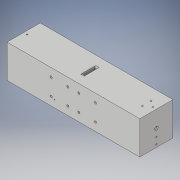
# Autodesk Inventor part: block
Saved by Autodesk Inventor 2017 (Build 210142000, 142)
## iProperties
Created: 2017-11-18
Part Number: block
Material: Generic
Document SubType Name: Modeling
Designer: Andy
Density: 1 g/cm^3
Appearance: Default
Author: Andy
Autodesk Inventor part; units mm, degrees
ref_plane "YZ Plane" through (0, 0, 0) normal (1, 0, 0) x (0, 1, 0)
ref_plane "XZ Plane" through (0, 0, 0) normal (0, 1, 0) x (-1, 0, 0)
ref_plane "XY Plane" through (0, 0, 0) normal (0, 0, 1) x (1, 0, 0)
sketch "Sketch1" plane through (0, 0, 0) normal (0, 0, 1) x (1, 0, 0)
  line L0 (-395.4763, 28.0534) -> (214.1237, 28.0534)
  line L1 (214.1237, 28.0534) -> (214.1237, -124.3466)
  line L2 (214.1237, -124.3466) -> (-395.4763, -124.3466)
  line L3 (-395.4763, -124.3466) -> (-395.4763, 28.0534)
  line L4 (100.4888, 124.4295) -> (100.4888, 286.3545)
  line L5 (100.4888, 286.3545) -> (135.4138, 286.3545)
  line L6 (137.9237, 286.3545) -> (137.9237, 124.4295)
  line L7 (137.9237, 124.4295) -> (100.4888, 124.4295)
  point P0 (0, 0)
  dimension "d0" = 609.6
  dimension "d1" = 152.4
  dimension "d7" = 161.925
  dimension "d8" = 34.925
  constraints: 16 end point, 3 perpendicular, 2 parallel, 2 vertical, 1 horizontal, 1 point on line
  measures "d0" distance between parallel lines of L1 L3
  measures "d1" distance between parallel lines of L2 L0
  measures "d7" distance of L4.start L4.end
  measures "d8" distance of L4.end L5.end
extrude "Extrusion1" add sketch "Sketch1" along normal blind 152.4
sketch "Sketch4" plane through (214.1237, -124.3466, 0) normal (1, 0, 0) x (0, 0, -1)
  circle A0 centre (-76.2, 76.2) radius 5.1594
  line L0 (-152.4, 0) -> (-152.4, 152.4) projected
  line L1 (0, 152.4) -> (-152.4, 152.4) projected
  point P0 (0, 124.3466)
  dimension "d1" = 152.4
  dimension "d9" = 10.3187
  constraints: 1 centre point
  measures "d9" diameter of A0
extrude "Extrusion2" cut sketch "Sketch4" against normal blind 609.6
sketch "Sketch5" plane through (-395.4763, 28.0534, 0) normal (0, 1, 0) x (1, 0, 0)
  line L0 (609.6, -152.4) -> (0, -152.4) projected
  line L1 (0, -152.4) -> (0, 0) projected
  line L2 (0, 0) -> (609.6, 0) projected
  line L3 (609.6, 0) -> (609.6, -152.4) projected
  line L4 (609.6, -152.4) -> (0, -152.4) projected
  line L5 (609.6, 0) -> (609.6, -152.4) projected
  line L6 (0, 0) -> (0, -152.4) projected
  line L7 (0, 0) -> (609.6, 0) projected
  line L8 (297.18, -104.775) -> (312.42, -104.775)
  line L9 (312.42, -104.775) -> (312.42, -47.625)
  line L10 (312.42, -47.625) -> (297.18, -47.625)
  line L11 (297.18, -47.625) -> (297.18, -104.775)
  line L12 (297.18, -104.775) -> (312.42, -47.625) construction
  line L13 (312.42, -104.775) -> (297.18, -47.625) construction
  point P0 (395.4763, 0)
  point P1 (297.0135, -78.1466)
  point P2 (312.2535, -78.0634)
  point P3 (312.2535, -74.3366)
  point P4 (304.8, -76.2)
  dimension "d1" = 152.4
  dimension "d48" = 15.24
  dimension "d49" = 57.15
  dimension "d50" = 47.625
  dimension "d51" = 47.625
  constraints: 12 end point, 2 midpoint, 2 parallel, 1 horizontal, 1 perpendicular
  measures "d48" distance of L10.end L9.end
  measures "d49" distance between parallel lines of L8 L10
  measures "d50" distance between parallel lines of L2 L10
  measures "d51" distance between parallel lines of L0 L8
extrude "Extrusion3" cut sketch "Sketch5" against normal blind 609.6 contours L11 L10 L9 L8
fillet "Fillet1" radius 6.35 4 edges at (-90.6763, 28.0534, 47.625) (-90.6763, 28.0534, 104.775) (-90.6763, -124.3466, 47.625) (-90.6763, -124.3466, 104.775)
chamfer "Chamfer1" distance 3.175 angle 45 1 edges at (214.1237, -48.1466, 81.3594) measured on face at (16.0037, -48.5618, 71.0574)
chamfer "Chamfer2" distance 3.175 angle 45 1 edges at (-395.4763, -48.1466, 81.3594) measured on face at (-296.4163, -48.5618, 71.0574)
sketch "Sketch6" plane through (-395.4763, 28.0534, 0) normal (0, 1, 0) x (1, 0, 0)
  line L0 (609.6, 0) -> (609.6, -152.4) projected
  line L1 (609.6, -152.4) -> (0, -152.4) projected
  line L2 (0, -152.4) -> (0, 0) projected
  line L3 (0, 0) -> (609.6, 0) projected
  line L4 (609.6, -84.5344) -> (609.6, -67.8656) projected
  line L5 (609.6, -76.2) -> (625.475, -76.2) construction
  circle A0 centre (593.725, -76.2) radius 3.175
  line L6 (0, 0) -> (0, -152.4) projected
  circle A1 centre (15.875, -76.2) radius 3.175
  line L7 (297.18, -41.275) -> (312.42, -41.275) projected
  line L8 (312.42, -111.125) -> (312.42, -41.275) projected
  line L9 (312.42, -111.125) -> (297.18, -111.125) projected
  line L10 (297.18, -41.275) -> (297.18, -111.125) projected
  point P0 (395.4763, 0)
  dimension "d1" = 152.4
  dimension "d30" = 6.35
  dimension "d34" = 6.35
  constraints: 2 centre point, 2 end point, 1 horizontal, 1 midpoint
  measures "d30" diameter of A0
  measures "d34" diameter of A1
extrude "Extrusion4" cut sketch "Sketch6" against normal blind 101.6 contours A0 | A1
sketch "Sketch7" plane through (-395.4763, 28.0534, 0) normal (0, 1, 0) x (1, 0, 0)
  circle A0 centre (593.725, -76.2) radius 3.175 construction
  circle A1 centre (15.875, -76.2) radius 3.175 projected
  line L0 (609.6, 0) -> (609.6, -152.4) construction
  line L1 (609.6, -152.4) -> (0, -152.4) projected
  line L2 (0, -152.4) -> (0, 0) projected
  line L3 (0, 0) -> (609.6, 0) projected
  line L4 (609.6, -152.4) -> (0, -152.4) projected
  line L5 (565.15, -152.4) -> (565.15, 0) construction
  line L6 (609.6, 0) -> (609.6, -152.4) construction
  line L7 (297.18, -41.275) -> (312.42, -41.275) projected
  line L8 (312.42, -111.125) -> (312.42, -41.275) projected
  line L9 (312.42, -111.125) -> (297.18, -111.125) projected
  line L10 (297.18, -41.275) -> (297.18, -111.125) projected
  line L11 (609.6, -76.2) -> (629.3437, -76.2) construction
  line L12 (629.3437, -56.1975) -> (609.6, -56.1975) construction
  line L13 (629.3437, -96.2025) -> (609.6, -96.2025) construction
  line L14 (609.6, -96.2025) -> (529.5756, -96.2025) construction
  line L15 (609.6, -56.1975) -> (531.5543, -56.1975) construction
  circle A2 centre (565.15, -96.2025) radius 3.175
  circle A3 centre (565.15, -56.1975) radius 3.175
  point P0 (395.4763, 0)
  dimension "d1" = 152.4
  dimension "d37" = 44.45
  dimension "d85" = 20.0025
  dimension "d86" = 40.005
  dimension "d87" = 6.35
  dimension "d88" = 6.35
  dimension "d89" = 44.45
  constraints: 12 end point, 6 point on line, 3 horizontal, 2 centre point, 1 midpoint, 1 vertical
  measures "d37" distance between parallel lines of L5 L0
  measures "d85" distance between parallel lines of L11 L12
  measures "d86" distance between parallel lines of L12 L13
  measures "d87" diameter of A2
  measures "d88" diameter of A3
  measures "d89" distance from line of A2.centre L0
extrude "Extrusion5" cut sketch "Sketch7" against normal blind 28.575 contours A2 | A3
sketch "Sketch9" plane through (-395.4763, -124.3466, 0) normal (0, -1, 0) x (1, 0, 0)
  line L0 (609.6, 152.4) -> (609.6, 0) projected
  line L1 (609.6, 0) -> (0, 0) projected
  line L2 (0, 0) -> (0, 152.4) projected
  line L3 (0, 152.4) -> (609.6, 152.4) projected
  line L4 (312.42, 41.275) -> (297.18, 41.275) projected
  line L5 (297.18, 111.125) -> (297.18, 41.275) projected
  line L6 (297.18, 111.125) -> (312.42, 111.125) projected
  line L7 (312.42, 41.275) -> (312.42, 111.125) projected
  line L8 (0, 76.2) -> (609.6, 76.2) construction
  circle A0 centre (218.44, 76.2) radius 19.685
  point P0 (395.4763, 0)
  dimension "d1" = 152.4
  dimension "d65" = 39.37
  dimension "d66" = 78.74
  dimension "d69" = 0
  constraints: 2 end point, 2 midpoint, 1 centre point
  measures "d65" diameter of A0
  measures "d66" distance from line of L5 A0.centre
  measures "d69" distance from line of L8 A0.centre
extrude "Extrusion8" cut sketch "Sketch9" against normal blind 63.5 contours A0
sketch "Sketch10" plane through (0, 0, 152.4) normal (0, 0, 1) x (1, 0, 0)
  line L0 (214.1237, 28.0534) -> (214.1237, -124.3466) projected
  line L1 (214.1237, -124.3466) -> (-395.4763, -124.3466) projected
  line L2 (-395.4763, -124.3466) -> (-395.4763, 28.0534) projected
  line L3 (-395.4763, 28.0534) -> (214.1237, 28.0534) projected
  line L4 (-157.3513, -124.3466) -> (-196.7213, -124.3466) projected
  line L5 (-157.3513, -60.8466) -> (-196.7213, -60.8466) projected
  line L6 (-157.3513, -124.3466) -> (-196.7213, -124.3466) projected
  line L7 (-157.3513, -92.075) -> (-196.7213, -92.075)
  line L8 (-177.0363, -92.075) -> (-177.0363, -60.8466)
  point P0 (0, 0)
  dimension "d1" = 152.4
  dimension "d72" = 31.2284
  constraints: 4 end point, 2 midpoint, 1 parallel
  measures "d72" distance between parallel lines of L5 L7
hole "Hole1" at (-177.0363, -92.075, 152.4) direction (0, 0, -1) diameter 3.9624 depth 13.6144 tip angle 118 thread size "10-32 UNF" class "2B" standard "ANSI Unified Screw Threads"
sketch "Sketch11" plane through (214.1237, -124.3466, 0) normal (1, 0, 0) x (0, 0, -1)
  circle A0 centre (-76.2, 12.7) radius 3.175 projected
  circle A1 centre (-76.2, 42.0133) radius 3.175 projected
  point P0 (0, 124.3466)
  dimension "d1" = 152.4
extrude "Extrusion9" cut sketch "Sketch11" against normal blind 28.575
thread "Thread7" size "1/4-20 UNC" class "2B" standard "ANSI Unified Screw Threads" full length
thread "Thread8" size "1/4-20 UNC" class "2B" standard "ANSI Unified Screw Threads" full length
sketch "Sketch12" plane through (0, 0, 0) normal (0, 0, -1) x (-1, 0, 0)
  line L0 (-214.1237, -124.3466) -> (-214.1237, 28.0534) construction
  line L1 (-214.1237, 28.0534) -> (395.4763, 28.0534) construction
  line L2 (395.4763, 28.0534) -> (395.4763, -124.3466) construction
  line L3 (395.4763, -124.3466) -> (-214.1237, -124.3466) construction
  line L4 (90.6763, 28.0534) -> (90.6763, -124.3466) construction
  line L5 (392.3013, -42.9872) -> (392.3013, -53.306) projected
  line L6 (-36.3237, -111.6466) -> (90.6763, -111.6466) construction
  line L7 (90.6763, -111.6466) -> (90.6763, 15.3534) construction
  line L8 (90.6763, 15.3534) -> (-36.3237, 15.3534) construction
  line L9 (-36.3237, 15.3534) -> (-36.3237, -111.6466) construction
  line L10 (118.2888, 15.3534) -> (-69.9987, 15.3534) construction
  line L11 (118.2888, -10.0466) -> (-69.9987, -10.0466) construction
  line L12 (65.2763, 28.0534) -> (65.2763, -124.3466) construction
  circle A0 centre (65.2763, -10.0466) radius 4.7625
  circle A1 centre (-10.9237, -10.0466) radius 4.7625
  circle A2 centre (65.2763, -86.2466) radius 4.7625
  circle A3 centre (-10.9237, -86.2466) radius 4.7625
  line L13 (63.0639, -10.0466) -> (251.3514, -10.0466) construction
  line L14 (116.0763, 28.0534) -> (116.0763, -124.3466) construction
  circle A4 centre (116.0763, -10.0466) radius 4.7625
  circle A5 centre (192.2763, -10.0466) radius 4.7625
  circle A6 centre (116.0763, -86.2466) radius 4.7625
  circle A7 centre (192.2763, -86.2466) radius 4.7625
  point P0 (0, 0)
  point P1 (181.3527, 0)
  dimension "d1" = 152.4
  dimension "d97" = 127
  dimension "d98" = 127
  dimension "d99" = 25.4
  dimension "d100" = 25.4
  dimension "d101" = 9.525
  dimension "d104" = 76.2
  dimension "d107" = 76.2
  constraints: 20 end point, 9 symmetric about line, 8 centre point, 5 point on line, 4 parallel, 2 horizontal, 2 midpoint, 1 perpendicular, 1 vertical, 10 other
  measures "d97" distance of L8.end L7.end
  measures "d98" distance of L7.end L6.end
  measures "d99" distance between parallel lines of L10 L11
  measures "d100" distance between parallel lines of L4 L12
  measures "d101" diameter of A0
  measures "d104" distance of A0.centre A1.centre
  measures "d107" distance of A0.centre A2.centre
extrude "Extrusion10" cut sketch "Sketch12" against normal through all
body "Solid1"
